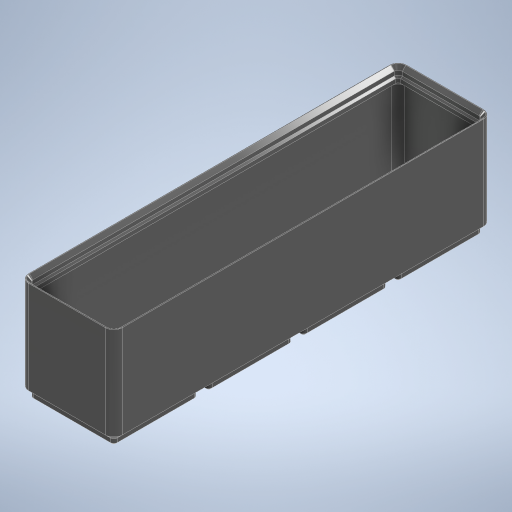
# Autodesk Inventor part: 4x1-bin-stackable
Saved by Autodesk Inventor 2023 (Build 270158030, 158C)
## iProperties
Created: 2023-12-22
Part Number: 4x1-bin-stackable
Material: Generic
Document SubType Name: Modeling
Designer: Imogen Heard
Density: 1 g/cm^3
Appearance: Dark Gray
Author: Imogen Heard
Autodesk Inventor part; units mm, degrees
ref_plane "YZ Plane" through (0, 0, 0) normal (1, 0, 0) x (0, 1, 0)
ref_plane "XZ Plane" through (0, 0, 0) normal (0, 1, 0) x (-1, 0, 0)
ref_plane "XY Plane" through (0, 0, 0) normal (0, 0, 1) x (1, 0, 0)
sketch "Sketch9" plane through (0, 0, 0) normal (0, 1, 0) x (-1, 0, 0)
  line L0 (-3.75, -41.5) -> (-37.75, -41.5)
  line L1 (-41.5, -37.75) -> (-41.5, -3.75)
  line L2 (-37.75, 0) -> (-3.75, 0)
  line L3 (0, -3.75) -> (0, -37.75)
  arc A0 (0, -3.75) -> (-3.75, 0) centre (-3.75, -3.75) ccw
  arc A1 (-37.75, 0) -> (-41.5, -3.75) centre (-37.75, -3.75) ccw
  arc A2 (-41.5, -37.75) -> (-37.75, -41.5) centre (-37.75, -37.75) ccw
  arc A3 (-3.75, -41.5) -> (0, -37.75) centre (-3.75, -37.75) ccw
  point P0 (0, 0)
  point P1 (0, -41.5)
  point P2 (-41.5, 0)
  point P3 (-41.5, -41.5)
  point P4 (0, 0)
  dimension "d50" = 41.5
  dimension "d51" = 41.5
  dimension "d52" = 3.75
  dimension "d55" = 3.75
  constraints: 8 end point, 8 point on circle, 8 point on line, 8 tangent, 4 centre point, 2 equal radius, 2 parallel, 1 coincident, 1 horizontal, 1 perpendicular
  measures "d50" distance between parallel lines of L1 L3
  measures "d51" distance between parallel lines of L2 L0
  measures "d52" radius of A0
  measures "d55" radius of A1
extrude "base-generic" add sketch "Sketch9" along normal blind 2.25
sketch "Sketch10" plane through (0, 0, 0) normal (0, -1, 0) x (1, 0, 0)
  line L0 (3.75, 0) -> (37.75, 0) projected
  arc A0 (3.75, 0) -> (0, -3.75) centre (3.75, -3.75) ccw projected
  line L1 (0, -37.75) -> (0, -3.75) projected
  arc A1 (0, -37.75) -> (3.75, -41.5) centre (3.75, -37.75) ccw projected
  line L2 (37.75, -41.5) -> (3.75, -41.5) projected
  arc A2 (37.75, -41.5) -> (41.5, -37.75) centre (37.75, -37.75) ccw projected
  line L3 (41.5, -3.75) -> (41.5, -37.75) projected
  arc A3 (41.5, -3.75) -> (37.75, 0) centre (37.75, -3.75) ccw projected
extrude "Extrusion8" add sketch "Sketch10" along normal blind 2.15 draft -45
sketch "Sketch11" plane through (0, -2.15, 0) normal (0, -1, 0) x (1, 0, 0)
  line L0 (37.75, -39.35) -> (3.75, -39.35) projected
  arc A0 (37.75, -39.35) -> (39.35, -37.75) centre (37.75, -37.75) ccw projected
  line L1 (39.35, -3.75) -> (39.35, -37.75) projected
  arc A1 (39.35, -3.75) -> (37.75, -2.15) centre (37.75, -3.75) ccw projected
  line L2 (3.75, -2.15) -> (37.75, -2.15) projected
  arc A2 (3.75, -2.15) -> (2.15, -3.75) centre (3.75, -3.75) ccw projected
  line L3 (2.15, -37.75) -> (2.15, -3.75) projected
  arc A3 (2.15, -37.75) -> (3.75, -39.35) centre (3.75, -37.75) ccw projected
  point P0 (0, 0)
extrude "Extrusion9" add sketch "Sketch11" along normal blind 1.8
sketch "Sketch12" plane through (0, -3.95, 0) normal (0, -1, 0) x (1, 0, 0)
  line L0 (37.75, -2.15) -> (3.75, -2.15) projected
  arc A0 (3.75, -2.15) -> (2.15, -3.75) centre (3.75, -3.75) ccw projected
  line L1 (2.15, -3.75) -> (2.15, -37.75) projected
  arc A1 (2.15, -37.75) -> (3.75, -39.35) centre (3.75, -37.75) ccw projected
  line L2 (3.75, -39.35) -> (37.75, -39.35) projected
  arc A2 (37.75, -39.35) -> (39.35, -37.75) centre (37.75, -37.75) ccw projected
  line L3 (39.35, -37.75) -> (39.35, -3.75) projected
  arc A3 (39.35, -3.75) -> (37.75, -2.15) centre (37.75, -3.75) ccw projected
  point P0 (0, 0)
extrude "Extrusion10" add sketch "Sketch12" along normal blind 0.8 draft -45
sketch "Sketch13" plane through (0, -4.75, 0) normal (0, -1, 0) x (1, 0, 0)
  circle A0 centre (7.75, -7.75) radius 3.25
  circle A1 centre (33.75, -7.75) radius 3.25
  circle A2 centre (33.75, -33.75) radius 3.25
  circle A3 centre (7.75, -33.75) radius 3.25
  line L0 (0, -37.75) -> (0, -3.75) projected
  line L1 (3.75, 0) -> (37.75, 0) projected
  line L2 (37.75, -41.5) -> (3.75, -41.5) projected
  line L3 (41.5, -3.75) -> (41.5, -37.75) projected
  point P0 (0, 0)
  dimension "d62" = 6.5
  dimension "d63" = 7.75
  dimension "d64" = 7.75
  dimension "d65" = 7.75
  dimension "d66" = 7.75
  constraints: 4 centre point, 3 equal radius, 2 horizontal alignment, 2 vertical alignment
  measures "d62" diameter of A0
  measures "d63" distance from line of L0 A0.centre
  measures "d64" distance from line of L1 A0.centre
  measures "d65" distance from line of L2 A3.centre
  measures "d66" distance from line of L3 A1.centre
extrude "Extrusion11" cut sketch "Sketch13" against normal blind 2.4
sketch "Sketch14" plane through (0, -4.75, 0) normal (0, -1, 0) x (1, 0, 0)
  circle A0 centre (7.75, -7.75) radius 1.5
  circle A1 centre (33.75, -7.75) radius 1.5
  circle A2 centre (33.75, -33.75) radius 1.5
  circle A3 centre (7.75, -33.75) radius 1.5
  circle A4 centre (7.75, -7.75) radius 3.25 projected
  circle A5 centre (33.75, -7.75) radius 3.25 projected
  circle A6 centre (33.75, -33.75) radius 3.25 projected
  circle A7 centre (7.75, -33.75) radius 3.25 projected
  point P0 (0, 0)
  dimension "d69" = 3
  constraints: 4 centre point, 4 concentric, 3 equal radius
  measures "d69" diameter of A0
extrude "Extrusion12" cut sketch "Sketch14" against normal blind 6 contours A0 | A1 | A2 | A3
pattern_linear "Rectangular Pattern1" count 4 spacing 42 along (0, 0, -1)
sketch "Sketch15" plane through (-38.25, 2.25, 0) normal (0, 1, 0) x (1, 0, 0)
  line L0 (76, 167.5) -> (42, 167.5)
  line L1 (38.25, 163.75) -> (38.25, 3.75)
  line L2 (42, 0) -> (76, 0)
  line L3 (79.75, 3.75) -> (79.75, 163.75)
  arc A0 (42, 167.5) -> (38.25, 163.75) centre (42, 163.75) ccw
  arc A1 (79.75, 163.75) -> (76, 167.5) centre (76, 163.75) ccw
  arc A2 (76, 0) -> (79.75, 3.75) centre (76, 3.75) ccw
  arc A3 (38.25, 3.75) -> (42, 0) centre (42, 3.75) ccw
  point P0 (0, 83.5)
  point P1 (0, 0)
  point P2 (38.25, 0)
  point P3 (38.25, 167.5)
  point P4 (79.75, 0)
  point P5 (42, 167.5)
  point P6 (42, 0)
  point P7 (79.75, 3.75)
  point P8 (38.25, 3.75)
  dimension "d82" = 3.75
  constraints: 8 end point, 8 point on circle, 8 tangent, 6 point on line, 4 centre point, 3 equal radius, 2 horizontal alignment, 2 parallel, 2 vertical alignment, 1 horizontal, 1 perpendicular
  measures "d82" radius of A0
extrude "fill-gaps" add sketch "Sketch15" against normal blind 2.25
sketch "Sketch16" plane through (0, 2.25, 0) normal (0, 1, 0) x (1, 0, 0)
  line L0 (0, 163.75) -> (0, 3.75) projected
  arc A0 (0, 3.75) -> (3.75, 0) centre (3.75, 3.75) ccw projected
  line L1 (3.75, 0) -> (37.75, 0) projected
  arc A1 (37.75, 0) -> (41.5, 3.75) centre (37.75, 3.75) ccw projected
  line L2 (41.5, 3.75) -> (41.5, 163.75) projected
  arc A2 (41.5, 163.75) -> (37.75, 167.5) centre (37.75, 163.75) ccw projected
  line L3 (37.75, 167.5) -> (3.75, 167.5) projected
  arc A3 (3.75, 167.5) -> (0, 163.75) centre (3.75, 163.75) ccw projected
  point P0 (0, 0)
extrude "Extrusion14" add sketch "Sketch16" along normal blind 39.4
sketch "Sketch19" plane through (0, 41.65, 0) normal (0, 1, 0) x (1, 0, 0)
  arc A0 (0, 3.75) -> (3.75, 0) centre (3.75, 3.75) ccw projected
  line L0 (3.75, 0) -> (37.75, 0) projected
  arc A1 (37.75, 0) -> (41.5, 3.75) centre (37.75, 3.75) ccw projected
  line L1 (41.5, 3.75) -> (41.5, 163.75) projected
  arc A2 (41.5, 163.75) -> (37.75, 167.5) centre (37.75, 163.75) ccw projected
  line L2 (37.75, 167.5) -> (3.75, 167.5) projected
  arc A3 (3.75, 167.5) -> (0, 163.75) centre (3.75, 163.75) ccw projected
  line L3 (0, 163.75) -> (0, 3.75) projected
  point P0 (0, 0)
extrude "Extrusion15" cut sketch "Sketch19" against normal blind 1.9 draft -45
sketch "Sketch20" plane through (0, 39.75, 0) normal (0, 1, 0) x (1, 0, 0)
  line L0 (3.75, 1.9) -> (37.75, 1.9) projected
  arc A0 (37.75, 1.9) -> (39.6, 3.75) centre (37.75, 3.75) ccw projected
  line L1 (39.6, 3.75) -> (39.6, 163.75) projected
  arc A1 (39.6, 163.75) -> (37.75, 165.6) centre (37.75, 163.75) ccw projected
  line L2 (37.75, 165.6) -> (3.75, 165.6) projected
  arc A2 (3.75, 165.6) -> (1.9, 163.75) centre (3.75, 163.75) ccw projected
  line L3 (1.9, 163.75) -> (1.9, 3.75) projected
  arc A3 (1.9, 3.75) -> (3.75, 1.9) centre (3.75, 3.75) ccw projected
  point P0 (0, 0)
extrude "Extrusion16" cut sketch "Sketch20" against normal blind 1.8
sketch "Sketch21" plane through (0, 37.95, 0) normal (0, 1, 0) x (1, 0, 0)
  arc A0 (37.75, 1.9) -> (39.6, 3.75) centre (37.75, 3.75) ccw projected
  line L0 (39.6, 163.75) -> (39.6, 3.75) projected
  arc A1 (39.6, 163.75) -> (37.75, 165.6) centre (37.75, 163.75) ccw projected
  line L1 (3.75, 165.6) -> (37.75, 165.6) projected
  arc A2 (3.75, 165.6) -> (1.9, 163.75) centre (3.75, 163.75) ccw projected
  line L2 (1.9, 3.75) -> (1.9, 163.75) projected
  arc A3 (1.9, 3.75) -> (3.75, 1.9) centre (3.75, 3.75) ccw projected
  line L3 (37.75, 1.9) -> (3.75, 1.9) projected
  point P0 (0, 0)
extrude "Extrusion17" cut sketch "Sketch21" against normal blind 0.7 draft -45
sketch "Sketch22" plane through (0, 37.25, 0) normal (0, 1, 0) x (1, 0, 0)
  line L0 (3.75, 2.6) -> (37.75, 2.6) projected
  arc A0 (37.75, 2.6) -> (38.9, 3.75) centre (37.75, 3.75) ccw projected
  line L1 (38.9, 3.75) -> (38.9, 163.75) projected
  arc A1 (38.9, 163.75) -> (37.75, 164.9) centre (37.75, 163.75) ccw projected
  line L2 (37.75, 164.9) -> (3.75, 164.9) projected
  arc A2 (3.75, 164.9) -> (2.6, 163.75) centre (3.75, 163.75) ccw projected
  line L3 (2.6, 163.75) -> (2.6, 3.75) projected
  arc A3 (2.6, 3.75) -> (3.75, 2.6) centre (3.75, 3.75) ccw projected
  point P0 (0, 0)
extrude "Extrusion18" cut sketch "Sketch22" against normal blind 1.8
sketch "Sketch23" plane through (0, 35.45, 0) normal (0, 1, 0) x (1, 0, 0)
  arc A0 (37.75, 2.6) -> (38.9, 3.75) centre (37.75, 3.75) ccw projected
  line L0 (38.9, 163.75) -> (38.9, 3.75) projected
  arc A1 (38.9, 163.75) -> (37.75, 164.9) centre (37.75, 163.75) ccw projected
  line L1 (3.75, 164.9) -> (37.75, 164.9) projected
  arc A2 (3.75, 164.9) -> (2.6, 163.75) centre (3.75, 163.75) ccw projected
  line L2 (2.6, 3.75) -> (2.6, 163.75) projected
  arc A3 (2.6, 3.75) -> (3.75, 2.6) centre (3.75, 3.75) ccw projected
  line L3 (37.75, 2.6) -> (3.75, 2.6) projected
  point P0 (0, 0)
extrude "Extrusion19" cut sketch "Sketch23" against normal blind 1.8 draft 45
sketch "Sketch24" plane through (0, 33.65, 0) normal (0, 1, 0) x (1, 0, 0)
  line L0 (3.75, 0.8) -> (37.75, 0.8) projected
  arc A0 (37.75, 0.8) -> (40.7, 3.75) centre (37.75, 3.75) ccw projected
  line L1 (40.7, 3.75) -> (40.7, 163.75) projected
  arc A1 (40.7, 163.75) -> (37.75, 166.7) centre (37.75, 163.75) ccw projected
  line L2 (37.75, 166.7) -> (3.75, 166.7) projected
  arc A2 (3.75, 166.7) -> (0.8, 163.75) centre (3.75, 163.75) ccw projected
  line L3 (0.8, 163.75) -> (0.8, 3.75) projected
  arc A3 (0.8, 3.75) -> (3.75, 0.8) centre (3.75, 3.75) ccw projected
  point P0 (0, 0)
extrude "Extrusion20" cut sketch "Sketch24" against normal blind 33
fillet "Fillet4" radius 0.2 8 edges at (40.4017, 41.65, -1.0983) (41.5, 41.65, -83.75) (40.4017, 41.65, -166.4017) (20.75, 41.65, -167.5) (1.0983, 41.65, -166.4017) (0, 41.65, -83.75) (1.0983, 41.65, -1.0983) (20.75, 41.65, 0)
equation "\"d51\" = d50"
equation "\"d64\" = d63"
equation "\"d65\" = d63"
equation "\"d66\" = d63"
body "Solid2"
